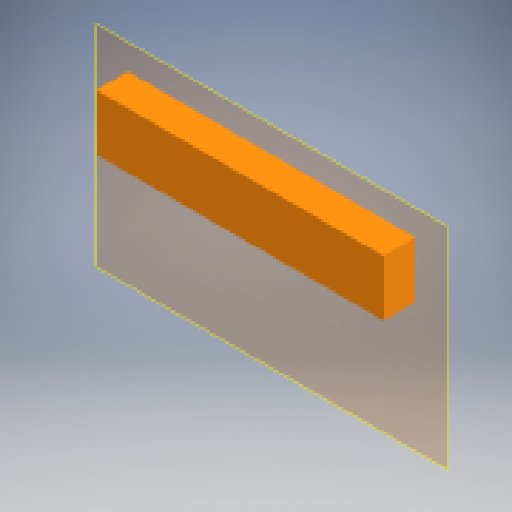
# Autodesk Inventor part: CE-8.2.2-01-003
Saved by Autodesk Inventor 2024 (Build 280153000, 153)
## iProperties
Created: 2024-03-07
Part Number: CE-8.2.2-01-003
Material: Generic
Document SubType Name: Modeling
Designer: Alex
Density: 1 g/cm^3
Appearance: Orange
Author: Alex
Autodesk Inventor part; units mm, degrees
ref_plane "YZ Plane" through (0, 0, 0) normal (1, 0, 0) x (0, 1, 0)
ref_plane "XZ Plane" through (0, 0, 0) normal (0, 1, 0) x (-1, 0, 0)
ref_plane "XY Plane" through (0, 0, 0) normal (0, 0, 1) x (1, 0, 0)
ref_plane "Work Plane1" through (50.0744, -24.8915, -44.5444) normal (0, 0, 1) x (1, 0, 0)
sketch "Sketch1" plane through (50.0744, -24.8915, -44.5444) normal (0, 0, 1) x (1, 0, 0)
  line L0 (10, 110) -> (190, 110)
  line L1 (10, 75) -> (10, 110)
  line L2 (190, 75) -> (10, 75)
  line L3 (190, 110) -> (190, 75)
  point P0 (-50.0744, 24.8915)
  constraints: 8 end point, 2 horizontal, 2 vertical, 4 other
extrude "Extrusion1" add sketch "Sketch1" along normal blind 20
body "Solid1"
